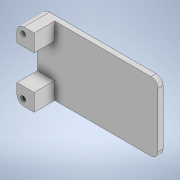
# Autodesk Inventor part: RDC1-0014_Holder
Saved by Autodesk Inventor 2020 (Build 240168000, 168)
## iProperties
Created: 2020-08-25
Part Number: RDC1-0014_Holder
Material: Типовые
Document SubType Name: Modeling
Designer: Михаил
Density: 1 g/cm^3
Appearance: По умолчанию
Author: Михаил
Autodesk Inventor part; units mm, degrees
ref_plane "YZ Plane" through (0, 0, 0) normal (1, 0, 0) x (0, 1, 0)
ref_plane "XZ Plane" through (0, 0, 0) normal (0, 1, 0) x (-1, 0, 0)
ref_plane "XY Plane" through (0, 0, 0) normal (0, 0, 1) x (1, 0, 0)
sketch "Эскиз1" plane through (0, 0, 0) normal (0, 0, 1) x (1, 0, 0)
  line L0 (0, 0) -> (35, 0)
  line L1 (35, 0) -> (35, 20)
  line L2 (35, 20) -> (0, 20)
  line L3 (0, 20) -> (0, 0)
  dimension "d0" = 35
  dimension "d1" = 20
  constraints: 8 end point, 2 parallel, 1 horizontal, 1 perpendicular
  measures "d0" distance of L2.end L1.end
  measures "d1" distance of L1.end L0.end
extrude "Выдавливание1" add sketch "Эскиз1" along normal blind 1.5
sketch "Эскиз2" plane through (0, 0, 1.5) normal (0, 0, 1) x (1, 0, 0)
  line L0 (0, 20) -> (0, 0) projected
  line L1 (0, 0) -> (5, 0)
  line L2 (5, 0) -> (5, 5)
  line L3 (5, 5) -> (0, 5)
  line L4 (0, 5) -> (0, 0)
  line L5 (35, 20) -> (0, 20) projected
  line L6 (0, 20) -> (5, 20)
  line L7 (5, 20) -> (5, 15)
  line L8 (5, 15) -> (0, 15)
  line L9 (0, 15) -> (0, 20)
  dimension "d4" = 5
  dimension "d5" = 5
  dimension "d6" = 5
  dimension "d7" = 5
  constraints: 16 end point, 4 parallel, 2 horizontal, 2 perpendicular
  measures "d4" distance of L7.end L8.end
  measures "d5" distance of L6.end L7.end
  measures "d6" distance of L2.end L3.end
  measures "d7" distance of L1.end L2.end
extrude "Выдавливание2" add sketch "Эскиз2" along normal blind 6
sketch "Эскиз3" plane through (0, 0, 7.5) normal (0, 0, 1) x (1, 0, 0)
  circle A0 centre (1.8, 1.8) radius 0.75
  circle A1 centre (1.8, 18.2) radius 0.75
  line L0 (0, 0) -> (5, 0) projected
  line L1 (0, 5) -> (0, 0) projected
  line L2 (0, 20) -> (0, 15) projected
  line L3 (5, 20) -> (0, 20) projected
  dimension "d10" = 1.5
  dimension "d11" = 1.5
  dimension "d12" = 1.8
  dimension "d13" = 1.8
  dimension "d14" = 1.8
  dimension "d15" = 1.8
  constraints: 2 centre point
  measures "d10" diameter of A0
  measures "d11" diameter of A1
  measures "d12" distance from line of L0 A0.centre
  measures "d13" distance from line of L1 A0.centre
  measures "d14" distance from line of L2 A1.centre
  measures "d15" distance from line of L3 A1.centre
extrude "Выдавливание3" cut sketch "Эскиз3" against normal blind 6
fillet "Сопряжение1" radius 2 4 edges at (0, 0, 3.75) (0, 20, 3.75) (35, 20, 0.75) (35, 0, 0.75)
